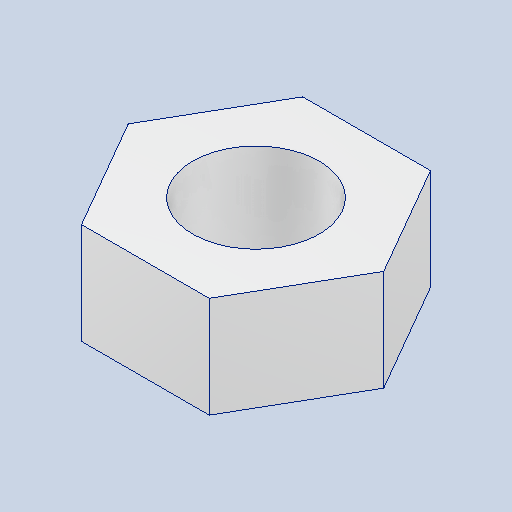
# Autodesk Inventor part: nat_M4
Saved by Autodesk Inventor 2024.1 (Build 281209000, 209)
## iProperties
Created: 2025-01-18
Part Number: nat_M4
Material: アルミニウム 6061
Document SubType Name: Modeling
Designer: hibik
Density: 2.7 g/cm^3
Appearance: アルミニウム - フラット
Author: hibik
Autodesk Inventor part; units mm, degrees
ref_plane "YZ Plane" through (0, 0, 0) normal (1, 0, 0) x (0, 1, 0)
ref_plane "XZ Plane" through (0, 0, 0) normal (0, 1, 0) x (-1, 0, 0)
ref_plane "XY Plane" through (0, 0, 0) normal (0, 0, 1) x (1, 0, 0)
sketch "スケッチ1" plane through (0, 0, 0) normal (0, 1, 0) x (-1, 0, 0)
  line L0 (-2.0207, 3.5) -> (2.0207, 3.5)
  line L1 (2.0207, 3.5) -> (4.0415, 0)
  line L2 (4.0415, 0) -> (2.0207, -3.5)
  line L3 (2.0207, -3.5) -> (-2.0207, -3.5)
  line L4 (-2.0207, -3.5) -> (-4.0415, 0)
  line L5 (-4.0415, 0) -> (-2.0207, 3.5)
  circle A0 centre (0, 0) radius 2
  dimension "d0" = 7
  dimension "d1" = 4
  constraints: 12 end point, 2 coincident, 1 centre point, 1 horizontal, 13 other
  measures "d0" distance between parallel lines of L4 L1
  measures "d1" diameter of A0
extrude "押し出し1" add sketch "スケッチ1" along normal blind 3.2
